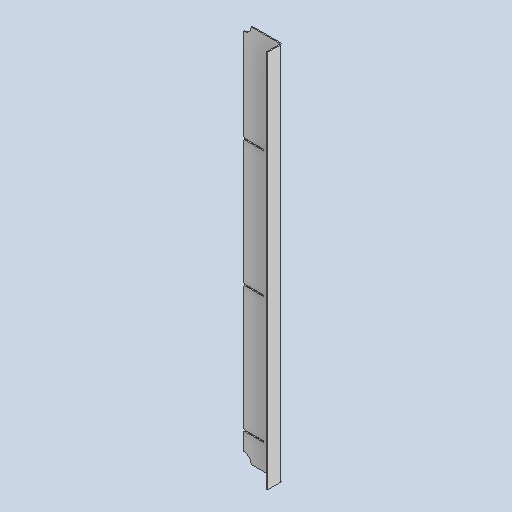
# Autodesk Inventor part: 0242 GBK stringer 5
Saved by Autodesk Inventor 2026 (Build 300175000, 175)
## iProperties
Created: 2026-05-07
Part Number: 0242 GBK stringer 5
Material: Steel
Document SubType Name: Sheet Metal
Designer: pokla
Density: 7.85 g/cm^3
Sheet Metal Rule: По умолчанию_мм
Appearance: Default
Author: admin
Autodesk Inventor part; units mm, degrees
ref_plane "YZ Plane" through (0, 0, 0) normal (1, 0, 0) x (0, 1, 0)
ref_plane "XZ Plane" through (0, 0, 0) normal (0, 1, 0) x (-1, 0, 0)
ref_plane "XY Plane" through (0, 0, 0) normal (0, 0, 1) x (1, 0, 0)
sketch "Sketch1" plane through (0, 0, 0) normal (0, 0, 1) x (1, 0, 0)
  line L0 (0, 0) -> (-145.2564, 0)
  line L1 (-145.2564, 0) -> (-145.2564, -1500)
  line L2 (-145.2564, -1500) -> (0, -1500)
  line L3 (0, -1500) -> (0, 0)
  line L4 (-145.2564, -1400) -> (-66, -1400)
  line L5 (-66, -1400) -> (-66, -1395)
  line L6 (-66, -1395) -> (-145.2564, -1395)
  line L7 (-145.2564, -1395) -> (-145.2564, -1400)
  line L8 (-145.2564, -900) -> (-66, -900)
  line L9 (-66, -900) -> (-66, -895)
  line L10 (-66, -895) -> (-145.2564, -895)
  line L11 (-145.2564, -895) -> (-145.2564, -900)
  line L12 (-145.2564, -400) -> (-66, -400)
  line L13 (-66, -400) -> (-66, -395)
  line L14 (-66, -395) -> (-145.2564, -395)
  line L15 (-145.2564, -395) -> (-145.2564, -400)
  circle A0 centre (-145.2564, 0) radius 30
  circle A1 centre (-145.2564, -1500) radius 30
  point P0 (-145.2564, -395)
  point P1 (-145.2564, -1395)
  point P2 (-115.2564, 0)
  point P3 (-145.2564, -30)
  point P4 (-145.2564, -1470)
  point P5 (-115.2564, -1500)
  dimension "d0" = 1500
  dimension "d1" = 145.2564
  dimension "d2" = 5
  dimension "d4" = 100
  dimension "d7" = 500
  dimension "d23" = 66
  dimension "d24" = 60
  measures "d0" distance of L1.end L0.end
  measures "d1" distance of L1.end L2.end
  measures "d2" distance of L4.end L5.end
  measures "d4" distance between parallel lines of L2 L4
  measures "d7" distance of L4.start L8.start
  measures "d23" distance between parallel lines of L3 L5
  measures "d24" diameter of A1
extrude "Plate1" add sketch "Sketch1" along normal blind 4 contours L3 L2 A1 L1 L4 L5 L6 L8 L9 L10 L12 L13 L14 A0 L0
sketch "Sketch2" plane through (4, 0, 0) normal (-1, 0, 0) x (0, -1, 0)
  line L0 (1500, 0) -> (0, 0)
  line L1 (0, 0) -> (0, 60)
  line L2 (0, 60) -> (1500, 60)
  line L3 (1500, 60) -> (1500, 0)
  constraints: 6 end point, 1 horizontal, 1 perpendicular, 1 vertical
edge flange "Flange1" height 60 angle 90 thickness 4 bend radius 4 thickness toward (-1, 0, 0) relief straight relief width 4 relief depth 2 edges at (0, -750, 4) wall of the first edge with corners at (4, -1500, 0) (4, 0, 0) (4, 0, 60) (4, -1500, 60)
bend "Bend1"
corner "Corner1"
chamfer "Corner Chamfer1" distance 3 angle 45 6 edges at (-145.2564, -1400, 2) (-145.2564, -1395, 2) (-145.2564, -900, 2) (-145.2564, -895, 2) (-145.2564, -395, 2) (-145.2564, -400, 2)
equation "\"d1\" = стрингер_глубина_5"
equation "\"d2\" = паз_под_стрингер_толщина"
equation "\"d23\" = паз_под_стрингер_глубина - Thickness"
equation "\"d24\" = 2 * радиус_выреза_под_сварку"
equation "\"d12\" = Thickness"
equation "\"d13\" = BendReliefWidth"
equation "\"d14\" = BendReliefDepth"
equation "\"d15\" = MinimumRemnant"
equation "\"d16\" = TransitionRadius"
equation "\"d17\" = ребро_усилителей"
equation "\"d19\" = BendRadius"
equation "\"d20\" = CornerReliefSize"
equation "\"d21\" = GapSize"
equation "\"d22\" = JacobiRadiusSize"
equation "\"BendRadius\" = Thickness"
equation "\"BendReliefWidth\" = Thickness"
equation "\"BendReliefDepth\" = 0.5 * Thickness"
equation "\"CornerReliefSize\" = 4 * Thickness"
equation "\"MinimumRemnant\" = 2 * Thickness"
equation "\"TransitionRadius\" = BendRadius"
equation "\"JacobiRadiusSize\" = BendRadius"
equation "\"GapSize\" = Thickness"
equation "\"стрингер_глубина_5\" = 145.256384"
equation "\"паз_под_стрингер_толщина\" = 5"
equation "\"паз_под_стрингер_глубина\" = 70"
equation "\"Thickness\" = 4"
equation "\"радиус_выреза_под_сварку\" = 30"
equation "\"ребро_усилителей\" = 60"
body "Solid1"
